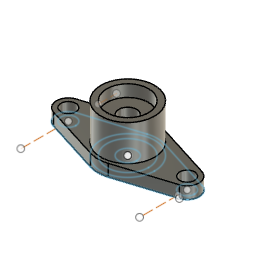
ex76 (Autodesk Fusion 360 design; units mm, degrees)
Autodesk Fusion 360 part; units mm, degrees
sketch "Sketch1" plane through (0, 0, 0) normal (0, 0, 1) x (1, 0, 0)
  circle A0 centre (0, 0) radius 15
  circle A1 centre (0, 0) radius 35
  circle A2 centre (0, 0) radius 45
  line L0 (-100, -20.9657) -> (-100, -80.0578) construction
  circle A3 centre (-100, 0) radius 12.5
  circle A4 centre (100, 0) radius 12.5
  line L1 (-106, 19.0788) -> (-15, 47.697)
  arc A5 (-106, 19.0788) -> (-106, -19.0788) centre (-100, 0) ccw
  line L2 (-106, -19.0788) -> (-15, -47.697)
  line L3 (106, 19.0788) -> (15, 47.697)
  line L4 (106, -19.0788) -> (15, -47.697)
  arc A6 (-15, -47.697) -> (15, -47.697) centre (0, 0) ccw
  arc A7 (15, 47.697) -> (-15, 47.697) centre (0, 0) ccw
  line L5 (100, -15) -> (100, -80.0578) construction
  line L6 (-100, 50) -> (-100, 80.9539) construction
  arc A8 (100, -20) -> (106, 19.0788) centre (100, 0) ccw
  dimension "d1" = 30
  dimension "d2" = 70
  dimension "d3" = 90
  dimension "d4" = 100
  dimension "d7" = 25
  dimension "d8" = 40
  constraint concentric A1 A2
  constraint concentric A3 A5
  constraint tangent L1 A6
  constraint tangent L1 A5
  constraint coincident L2 L0.start
  constraint concentric A6 A7
  constraint coincident L5 A8.start
  measures "d1" diameter of A0
  measures "d2" diameter of A1
  measures "d3" diameter of A2
  measures "d4" diameter of A6
  measures "d7" diameter of A3
  measures "d8" diameter of A5
extrude "Extrude1" add sketch "Sketch1" along normal blind 20 contours L1 A5 L2 L3 L4 A6 A7 A8
extrude "Extrude2" add sketch "Sketch1" along normal blind 80 contours A2
extrude "Extrude3" add sketch "Sketch1" along normal blind 60 contours A1
